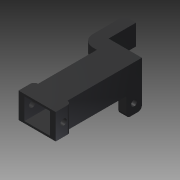
# Autodesk Inventor part: motoruchyt
Saved by Autodesk Inventor 2015 (Build 190159000, 159)
## iProperties
Created: 2015-05-23
Part Number: motoruchyt
Material: ABS Plastic
Document SubType Name: Modeling
Designer: Jufo
Density: 1 g/cm^3
Appearance: Smooth - White
Author: Jufo
Autodesk Inventor part; units mm, degrees
ref_plane "YZ Plane" through (0, 0, 0) normal (1, 0, 0) x (0, 1, 0)
ref_plane "XZ Plane" through (0, 0, 0) normal (0, 1, 0) x (-1, 0, 0)
ref_plane "XY Plane" through (0, 0, 0) normal (0, 0, 1) x (1, 0, 0)
sketch "Sketch1" plane through (0, 0, 0) normal (0, 1, 0) x (-1, 0, 0)
  line L0 (0, 6.5) -> (-5.5, 6.5)
  line L1 (-5.5, 6.5) -> (-5.5, -4.5)
  line L2 (-5.5, -4.5) -> (7.5, -4.5)
  line L3 (7.5, -4.5) -> (7.5, 6.5)
  line L4 (7.5, 6.5) -> (0, 6.5)
  line L5 (8.5, 7.5) -> (8.5, -5.5)
  line L6 (8.5, -5.5) -> (-6.5, -5.5)
  line L7 (-6.5, -5.5) -> (-6.5, 7.5)
  line L8 (-6.5, 7.5) -> (8.5, 7.5)
  point P0 (0, 0)
  dimension "d2" = 11
  dimension "d3" = 13
  dimension "d6" = 13
  dimension "d7" = 15
  dimension "d47" = 1
  dimension "d48" = 1
  constraints: 18 end point, 5 perpendicular, 1 collinear, 1 parallel
  measures "d2" distance of L0.end L1.end
  measures "d3" distance of L1.end L2.end
  measures "d6" distance of L5.start L5.end
  measures "d7" distance of L5.end L6.end
  measures "d47" distance between parallel lines of L8 L0
  measures "d48" distance between parallel lines of L1 L7
extrude "Extrusion1" add sketch "Sketch1" along normal blind 45
sketch "Sketch2" plane through (0, 45, 0) normal (0, 1, 0) x (1, 0, 0)
  line L0 (-8.5, 5.5) -> (-8.5, -7.5) projected
  line L1 (-8.5, -7.5) -> (6.5, -7.5) projected
  line L2 (6.5, -7.5) -> (6.5, 5.5) projected
  line L3 (6.5, 5.5) -> (-8.5, 5.5) projected
  circle A0 centre (0, 0) radius 2.5
  circle A1 centre (-4, 0) radius 0.75
  circle A2 centre (4, 0) radius 0.75
  dimension "d10" = 5
  dimension "d14" = 1.5
  constraints: 3 centre point, 1 coincident
  measures "d10" diameter of A0
  measures "d14" diameter of A1
extrude "Extrusion2" add sketch "Sketch2" along normal blind 1
sketch "Sketch3" plane through (6.5, 0, 7.5) normal (1, 0, 0) x (0, 0, -1)
  line L0 (0, 46) -> (13, 46) projected
  line L1 (0, 0) -> (0, 46) projected
  line L2 (6.5, 46) -> (6.5, 4)
  circle A0 centre (6.5, 4) radius 1.6
  point P0 (7.5, 0)
  dimension "d17" = 42
  dimension "d18" = 3.2
  constraints: 2 end point, 1 centre point, 1 coincident, 1 midpoint, 1 parallel
  measures "d17" distance of L2.start L2.end
  measures "d18" diameter of A0
extrude "Extrusion3" cut sketch "Sketch3" against normal blind 50
sketch "Sketch7" plane through (6.5, 0, -5.5) normal (0, 0, -1) x (-1, 0, 0)
  line L0 (0, 43) -> (0, 46)
  line L1 (0, 46) -> (4, 46)
  line L2 (4, 46) -> (4, 38)
  line L3 (4, 38) -> (0, 38)
  line L4 (0, 38) -> (0, 43)
  line L5 (11, 46) -> (11, 38)
  line L6 (11, 38) -> (15, 38)
  line L7 (15, 38) -> (15, 46)
  line L8 (15, 46) -> (11, 46)
  line L9 (0, 0) -> (0, 46) projected
  line L10 (0, 46) -> (15, 46) projected
  point P0 (6.5, 0)
  dimension "d33" = 3
  dimension "d34" = 8
  dimension "d35" = 7
  dimension "d36" = 4
  dimension "d37" = 4
  dimension "d38" = 8
  dimension "d55" = 0
  dimension "d92" = 7
  dimension "d93" = 0
  constraints: 18 end point, 4 perpendicular, 1 collinear, 1 parallel, 1 point on line
  measures "d33" distance of L0.start L0.end
  measures "d34" distance of L1.end L2.end
  measures "d35" distance of L1.end L5.start
  measures "d36" distance of L0.end L1.end
  measures "d37" distance of L5.end L6.end
  measures "d38" distance of L5.start L5.end
  measures "d55" distance between parallel lines of L9 L4
  measures "d92" distance of L5.end L2.end
  measures "d93" distance between parallel lines of L10 L1
extrude "Extrusion7" add sketch "Sketch7" along normal blind 10
sketch "Sketch9" plane through (0, 46, 0) normal (0, 1, 0) x (1, 0, 0)
  circle A0 centre (0, 0) radius 2.5 projected
  circle A1 centre (4, 0) radius 0.75 projected
  circle A2 centre (-4, 0) radius 0.75 projected
  circle A3 centre (-4, 0) radius 0.75
  circle A4 centre (4, 0) radius 0.75
  circle A5 centre (0, 0) radius 2.5
  constraints: 3 centre point, 3 coincident, 3 concentric
extrude "Extrusion9" add sketch "Sketch9" against normal blind 1
sketch "Sketch11" plane through (0, 46, 0) normal (0, 1, 0) x (1, 0, 0)
  line L0 (2.5, 5.5) -> (-4.5, 5.5) projected
  line L1 (6.5, 5.5) -> (-1, 5.5)
  line L2 (-1, 5.5) -> (-1, -1)
  circle A0 centre (-1, -1) radius 2.5
  point P0 (-17.5, 5.5)
  point P1 (0, 0)
  point P2 (-18.5, 5.5)
  point P3 (-8.5, 5.5)
  dimension "d51" = 7.5
  dimension "d52" = 5
  constraints: 4 end point, 1 centre point, 1 coincident, 1 midpoint, 1 perpendicular
  measures "d51" distance of L1.start L1.end
  measures "d52" diameter of A0
extrude "Extrusion10" cut sketch "Sketch11" against normal blind 1
sketch "Sketch12" plane through (6.5, 0, 7.5) normal (1, 0, 0) x (0, 0, -1)
  circle A0 centre (18.05, 42) radius 1.5
  line L0 (13, 38) -> (23, 38) projected
  line L1 (0, 46) -> (23, 46) projected
  point P0 (7.5, 0)
  dimension "d56" = 3
  dimension "d104" = 4
  dimension "d105" = 4
  constraints: 1 centre point
  measures "d56" diameter of A0
  measures "d104" distance from line of L1 A0.centre
  measures "d105" distance from line of L0 A0.centre
extrude "Extrusion11" cut sketch "Sketch12" against normal blind 15
sketch "Sketch16" plane through (-8.5, 39, -13.5) normal (-1, 0, 0) x (0, 0, 1)
  line L0 (9, -34) -> (9, -2) projected
  line L1 (21, -39) -> (8, -39) projected
  line L2 (20, 3) -> (20, -34) projected
  circle A0 centre (14.5, -35) radius 1.6 projected
  line L3 (8, -39) -> (8, -1) projected
  line L4 (21, -39) -> (21, 7) projected
  line L5 (8, -31) -> (21, -31)
  point P0 (13.5, -39)
  point P1 (9, -26)
  point P2 (20, -26)
  point P3 (21, 6)
  point P4 (21, 3)
  point P5 (21, 5)
  point P6 (14.5, -39)
  dimension "d94" = 8
  constraints: 4 point on line, 2 end point, 1 perpendicular, 2 other
extrude "Extrusion15" add sketch "Sketch16" along normal blind 2
sketch "Sketch17" plane through (6.5, 0, 7.5) normal (1, 0, 0) x (0, 0, -1)
  circle A0 centre (6.5, 4) radius 1.6 projected
  line L0 (13, 0) -> (0, 0) projected
  line L1 (13, 0) -> (0, 0) projected
  line L2 (13, 0) -> (13, 38) projected
  line L3 (0, 45) -> (23, 45) projected
  line L4 (6.5, 0) -> (6.5, 8)
  line L5 (-8, 0) -> (13, 0)
  line L6 (0, 0) -> (0, 46) projected
  line L7 (0, 8) -> (13, 8)
  point P0 (19, 45)
  point P1 (7.5, 0)
  point P2 (23, 46)
  dimension "d78" = 8
  constraints: 6 end point, 4 point on line, 2 perpendicular, 1 midpoint, 1 vertical, 1 other
  measures "d78" distance of L4.start L4.end
fillet "Fillet11" radius 2 4 edges at (4.5, 46, -15.5) (4.5, 38, -15.5) (-6.5, 46, -15.5) (-6.5, 38, -15.5)
extrude "Extrusion18" add sketch "Sketch17" along normal blind 2 contours A0 L4 L7 L2 L0 | A0 L4 L0 L6 L7
sketch "Sketch21" plane through (-8.5, 8, 7.5) normal (-1, 0, 0) x (0, 0, 1)
  line L0 (0, 0) -> (0, 38) projected
  line L1 (-13, 52) -> (0, 52)
  line L2 (0, 52) -> (0, 30)
  line L3 (-13, 52) -> (-13, 30)
  line L4 (-13, 30) -> (0, 30)
  point P0 (-7.5, -8)
  dimension "d130" = 22
  dimension "d131" = 22
  constraints: 8 end point, 1 parallel, 1 perpendicular, 1 point on line
  measures "d130" distance of L1.start L3.end
  measures "d131" distance of L1.end L2.end
extrude "Extrusion19" add sketch "Sketch21" along normal blind 8
fillet "Fillet16" radius 2 2 edges at (-10.5, 8, 1) (8.5, 8, 1)
sketch "Sketch23" plane through (-8.5, 38, -5.5) normal (-1, 0, 0) x (0, 0, 1)
  circle A0 centre (6.5, -18) radius 1.5
  line L0 (0, -30) -> (13, -30) projected
  point P0 (5.5, -38)
  dimension "d114" = 3
  dimension "d142" = 12
  constraints: 1 centre point
  measures "d114" diameter of A0
  measures "d142" distance from line of L0 A0.centre
extrude "Extrusion20" cut sketch "Sketch23" against normal blind 2
sketch "Sketch24" plane through (-16.5, 8, 7.5) normal (-1, 0, 0) x (0, 0, 1)
  line L0 (0, 52) -> (-13, 52) projected
  line L1 (-6.5, 52) -> (-7.5, 52)
  line L2 (-6.5, 52) -> (-5.5, 52)
  line L3 (-7.5, 52) -> (-7.5, 51)
  line L4 (-13, 30) -> (0, 30) projected
  line L5 (-7.5, 52) -> (-7.5, 30)
  line L6 (-5.5, 52) -> (-5.5, 30)
  line L7 (-13, 52) -> (-13, 30) projected
  line L8 (-7.5, 51) -> (-5.5, 51)
  point P0 (-7.5, -8)
  dimension "d117" = 1
  dimension "d118" = 1
  dimension "d119" = 1
  constraints: 12 end point, 5 point on line, 3 perpendicular, 1 midpoint
  measures "d117" distance of L1.start L1.end
  measures "d118" distance of L1.start L2.end
  measures "d119" distance of L1.end L3.end
sketch "Sketch25" plane through (-16.5, 8, 7.5) normal (-1, 0, 0) x (0, 0, 1)
  line L0 (0, 52) -> (-13, 52) projected
  line L1 (-13, 52) -> (-13, 30) projected
  line L2 (-6.5, 52) -> (-10.5, 52)
  line L3 (-10.5, 52) -> (-10.5, 31)
  line L4 (-6.5, 52) -> (-2.5, 52)
  line L5 (-2.5, 52) -> (-2.5, 31)
  line L6 (-13, 30) -> (0, 30) projected
  line L7 (-10.5, 31) -> (-10.5, 30)
  line L8 (-2.5, 31) -> (-2.5, 30)
  point P0 (-7.5, -8)
  dimension "d122" = 4
  dimension "d123" = 4
  dimension "d129" = 22
  constraints: 12 end point, 4 point on line, 2 perpendicular, 1 midpoint, 1 parallel
  measures "d122" distance of L2.start L2.end
  measures "d123" distance of L2.start L4.end
  measures "d129" distance of L0.end L1.end
extrude "Extrusion22" cut sketch "Sketch24" against normal blind 4 contours L6 L4 L5 L8
fillet "Fillet17" radius 6 2 edges at (-16.5, 38, -2.75) (-16.5, 38, 4.75)
chamfer "Chamfer1" distance 2 angle 45 1 edges at (-12.5, 38.3431, 1)
sketch "Sketch26" plane through (-16.5, 8, 7.5) normal (-1, 0, 0) x (0, 0, 1)
  line L0 (-2.5, 36) -> (-5.5, 36) projected
  line L1 (-7.5, 36) -> (-7.5, 51) projected
  line L2 (-5.5, 51) -> (-5.5, 36) projected
  line L3 (-7.5, 36) -> (-5.5, 36)
  line L4 (-7.5, 51) -> (-7.5, 40)
  line L5 (-7.5, 40) -> (-5.5, 40)
  point P0 (-7.5, -8)
  dimension "d135" = 11
  constraints: 6 end point, 2 point on line, 1 collinear, 1 perpendicular
  measures "d135" distance of L1.end L4.end
extrude "Extrusion24" add sketch "Sketch26" against normal blind 2
extrude "Extrusion25" cut sketch "Sketch25" against normal blind 8 contours L3 L7 L6 L1 L0
sketch "Sketch27" plane through (-8.5, 8, 7.5) normal (1, 0, 0) x (0, 0, -1)
  line L0 (10.5, 38) -> (10.5, 52) projected
  line L1 (0, 52) -> (10.5, 52) projected
  line L2 (0, 38) -> (0, 52) projected
  line L3 (0, 38) -> (10.5, 38) projected
  point P0 (7.5, -8)
extrude "Extrusion26" cut sketch "Sketch27" against normal blind 2
body "Solid1"
